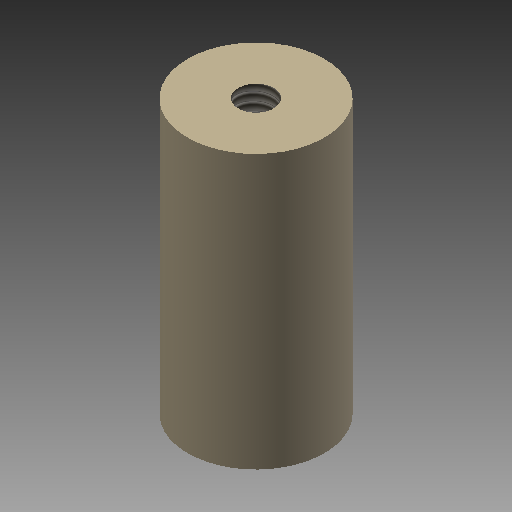
# Autodesk Inventor part: alumina_standoff_LSP_ASO00110
Saved by Autodesk Inventor 2018 (Build 220112000, 112)
## iProperties
Created: 2017-09-13
Part Number: alumina_standoff_LSP_ASO00110
Material: Generic
Document SubType Name: Modeling
Designer: pnigge
Density: 1 g/cm^3
Appearance: Beige
Author: pnigge
Autodesk Inventor part; units mm, degrees
ref_plane "YZ Plane" through (0, 0, 0) normal (1, 0, 0) x (0, 1, 0)
ref_plane "XZ Plane" through (0, 0, 0) normal (0, 1, 0) x (-1, 0, 0)
ref_plane "XY Plane" through (0, 0, 0) normal (0, 0, 1) x (1, 0, 0)
sketch "Sketch1" plane through (0, 0, 0) normal (0, 1, 0) x (-1, 0, 0)
  circle A0 centre (0, 0) radius 6.35
  dimension "d0" = 12.7
  constraints: 1 centre point, 1 coincident
  measures "d0" diameter of A0
extrude "Extrusion1" add sketch "Sketch1" along normal blind 25.4
hole "Hole1" at (0, 25.4, 0) direction (0, -1, 0) diameter 3.302 depth 9.525 tip angle 118 thread size "8-32 UNC" class "2B" standard "ANSI Unified Screw Threads"
hole "Hole2" at (0, 0, 0) direction (0, 1, 0) diameter 3.302 depth 9.525 tip angle 118 thread size "8-32 UNC" class "2B" standard "ANSI Unified Screw Threads"
body "Solid1"
